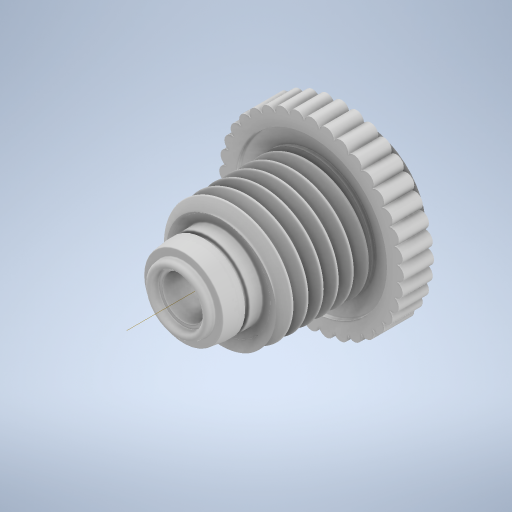
# Autodesk Inventor part: rosca
Saved by Autodesk Inventor 2024 (Build 280153000, 153)
## iProperties
Created: 2023-07-06
Part Number: rosca
Material: Genérico
Document SubType Name: Modeling
Designer: Arthur
Density: 1 g/cm^3
Appearance: Valor por defecto
Author: Arthur
## iProperties of the stored document rosca_3DPrint.ipt
Created: 2023-07-06
Part Number: rosca_3DPrint
Material: Genérico
Document SubType Name: Modeling
Designer: Arthur
Density: 1 g/cm^3
Appearance: Valor por defecto
Author: Arthur
Autodesk Inventor part; units mm, degrees
ref_plane "YZ Plane" through (0, 0, 0) normal (1, 0, 0) x (0, 1, 0)
ref_plane "XZ Plane" through (0, 0, 0) normal (0, 1, 0) x (-1, 0, 0)
ref_plane "XY Plane" through (0, 0, 0) normal (0, 0, 1) x (1, 0, 0)
sketch "Boceto1" plane through (0, 0, 0) normal (0, 0, 1) x (1, 0, 0)
  circle A0 centre (0, 0) radius 11.25
  arc A1 (0.999, 11.2056) -> (-0.999, 11.2056) centre (0, 11.25) ccw
  arc A2 (-0.962, 11.2088) -> (-2.9297, 10.8618) centre (-1.9535, 11.0791) ccw
  arc A3 (-2.8938, 10.8715) -> (-4.7713, 10.1881) centre (-3.8477, 10.5715) ccw
  arc A4 (-4.7376, 10.2038) -> (-6.4679, 9.2048) centre (-5.625, 9.7428) ccw
  arc A5 (-6.4375, 9.2261) -> (-7.9681, 7.9418) centre (-7.2314, 8.618) ccw
  arc A6 (-7.9418, 7.9681) -> (-9.2261, 6.4375) centre (-8.618, 7.2314) ccw
  arc A7 (-9.2048, 6.4679) -> (-10.2038, 4.7376) centre (-9.7428, 5.625) ccw
  arc A8 (-10.1881, 4.7713) -> (-10.8715, 2.8938) centre (-10.5715, 3.8477) ccw
  arc A9 (-10.8618, 2.9297) -> (-11.2088, 0.962) centre (-11.0791, 1.9535) ccw
  arc A10 (-11.2056, 0.999) -> (-11.2056, -0.999) centre (-11.25, 0) ccw
  arc A11 (-11.2088, -0.962) -> (-10.8618, -2.9297) centre (-11.0791, -1.9535) ccw
  arc A12 (-10.8715, -2.8938) -> (-10.1881, -4.7713) centre (-10.5715, -3.8477) ccw
  arc A13 (-10.2038, -4.7376) -> (-9.2048, -6.4679) centre (-9.7428, -5.625) ccw
  arc A14 (-9.2261, -6.4375) -> (-7.9418, -7.9681) centre (-8.618, -7.2314) ccw
  arc A15 (-7.9681, -7.9418) -> (-6.4375, -9.2261) centre (-7.2314, -8.618) ccw
  arc A16 (-6.4679, -9.2048) -> (-4.7376, -10.2038) centre (-5.625, -9.7428) ccw
  arc A17 (-4.7713, -10.1881) -> (-2.8938, -10.8715) centre (-3.8477, -10.5715) ccw
  arc A18 (-2.9297, -10.8618) -> (-0.962, -11.2088) centre (-1.9535, -11.0791) ccw
  arc A19 (-0.999, -11.2056) -> (0.999, -11.2056) centre (0, -11.25) ccw
  arc A20 (0.962, -11.2088) -> (2.9297, -10.8618) centre (1.9535, -11.0791) ccw
  arc A21 (2.8938, -10.8715) -> (4.7713, -10.1881) centre (3.8477, -10.5715) ccw
  arc A22 (4.7376, -10.2038) -> (6.4679, -9.2048) centre (5.625, -9.7428) ccw
  arc A23 (6.4375, -9.2261) -> (7.9681, -7.9418) centre (7.2314, -8.618) ccw
  arc A24 (7.9418, -7.9681) -> (9.2261, -6.4375) centre (8.618, -7.2314) ccw
  arc A25 (9.2048, -6.4679) -> (10.2038, -4.7376) centre (9.7428, -5.625) ccw
  arc A26 (10.1881, -4.7713) -> (10.8715, -2.8938) centre (10.5715, -3.8477) ccw
  arc A27 (10.8618, -2.9297) -> (11.2088, -0.962) centre (11.0791, -1.9535) ccw
  arc A28 (11.2056, -0.999) -> (11.2056, 0.999) centre (11.25, 0) ccw
  arc A29 (11.2088, 0.962) -> (10.8618, 2.9297) centre (11.0791, 1.9535) ccw
  arc A30 (10.8715, 2.8938) -> (10.1881, 4.7713) centre (10.5715, 3.8477) ccw
  arc A31 (10.2038, 4.7376) -> (9.2048, 6.4679) centre (9.7428, 5.625) ccw
  arc A32 (9.2261, 6.4375) -> (7.9418, 7.9681) centre (8.618, 7.2314) ccw
  arc A33 (7.9681, 7.9418) -> (6.4375, 9.2261) centre (7.2314, 8.618) ccw
  arc A34 (6.4679, 9.2048) -> (4.7376, 10.2038) centre (5.625, 9.7428) ccw
  arc A35 (4.7713, 10.1881) -> (2.8938, 10.8715) centre (3.8477, 10.5715) ccw
  arc A36 (2.9297, 10.8618) -> (0.962, 11.2088) centre (1.9535, 11.0791) ccw
  circle A37 centre (0, 0) radius 11.4037
  point P0 (-2.9515, 11.0151)
  point P1 (-4.8194, 10.3353)
  point P2 (-6.5409, 9.3414)
  point P3 (-8.0636, 8.0636)
  point P4 (-9.3414, 6.5409)
  point P5 (-10.3353, 4.8194)
  point P6 (-11.0151, 2.9515)
  point P7 (-11.3603, 0.9939)
  point P8 (-11.3603, -0.9939)
  point P9 (-11.0151, -2.9515)
  point P10 (-10.3353, -4.8194)
  point P11 (-9.3414, -6.5409)
  point P12 (-8.0636, -8.0636)
  point P13 (-6.5409, -9.3414)
  point P14 (-4.8194, -10.3353)
  point P15 (-2.9515, -11.0151)
  point P16 (-0.9939, -11.3603)
  point P17 (0.9939, -11.3603)
  point P18 (2.9515, -11.0151)
  point P19 (4.8194, -10.3353)
  point P20 (6.5409, -9.3414)
  point P21 (8.0636, -8.0636)
  point P22 (9.3414, -6.5409)
  point P23 (10.3353, -4.8194)
  point P24 (11.0151, -2.9515)
  point P25 (11.3603, -0.9939)
  point P26 (11.3603, 0.9939)
  point P27 (11.0151, 2.9515)
  point P28 (10.3353, 4.8194)
  point P29 (9.3414, 6.5409)
  point P30 (8.0636, 8.0636)
  point P31 (6.5409, 9.3414)
  point P32 (4.8194, 10.3353)
  point P33 (2.9515, 11.0151)
  point P34 (0.9939, 11.3603)
  point P35 (-0.9939, 11.3603)
  dimension "d1" = 22.5
  dimension "d4" = 360
  constraints: 75 point on circle, 38 centre point, 1 coincident, 145 other
  measures "d1" diameter of A0
extrude "Extrusión1" add sketch "Boceto1" along normal blind 4
sketch "Boceto2" plane through (0, 0, 0) normal (0, 0, -1) x (-1, 0, 0)
  circle A0 centre (0, 0) radius 8.25
  dimension "d8" = 16.5
  constraints: 1 centre point, 1 coincident
  measures "d8" diameter of A0
extrude "Extrusión2" add sketch "Boceto2" along normal blind 3
sketch "Boceto3" plane through (0, 0, 4) normal (0, 0, 1) x (1, 0, 0)
  circle A0 centre (0, 0) radius 8
  dimension "d11" = 16
  constraints: 1 centre point, 1 coincident
  measures "d11" diameter of A0
extrude "Extrusión3" add sketch "Boceto3" along normal blind 18
sketch "Boceto4" plane through (0, 0, 22) normal (0, 0, 1) x (1, 0, 0)
  circle A0 centre (0, 0) radius 8 projected
  circle A1 centre (0, 0) radius 5.5
  dimension "d14" = 11
  constraints: 1 centre point, 1 coincident
  measures "d14" diameter of A1
extrude "Extrusión4" cut sketch "Boceto4" against normal blind 6
sketch "Boceto5" plane through (0, 0, 22) normal (0, 0, 1) x (1, 0, 0)
  circle A0 centre (0, 0) radius 2.8
  dimension "d17" = 5.6
  constraints: 1 centre point, 1 coincident
  measures "d17" diameter of A0
extrude "Extrusión5" cut sketch "Boceto5" against normal blind 60
sketch "Boceto6" plane through (0, 0, 4) normal (0, 0, 1) x (1, 0, 0)
  circle A0 centre (0, 0) radius 10
  circle A1 centre (0, 0) radius 8
  circle A2 centre (0, 0) radius 8
  dimension "d20" = 20
  constraints: 3 centre point, 3 coincident
  measures "d20" diameter of A0
extrude "Extrusión6" cut sketch "Boceto6" against normal blind 0.5 contours A0 | A1
sketch "Boceto7" plane through (0, 0, 3.5) normal (0, 0, 1) x (1, 0, 0)
  circle A0 centre (0, 0) radius 8
  circle A1 centre (0, 0) radius 2.8
  constraints: 2 centre point, 2 coincident
extrude "Extrusión7" add sketch "Boceto7" along normal blind 0.5
sketch "Boceto8" plane through (0, 0, -3) normal (0, 0, -1) x (-1, 0, 0)
  circle A0 centre (0, 0) radius 2.8 projected
  circle A1 centre (0, 0) radius 5.4
  dimension "d27" = 10.8
  constraints: 1 centre point, 1 coincident
  measures "d27" diameter of A1
extrude "Extrusión8" cut sketch "Boceto8" against normal blind 10
fillet "Empalme1" radius 0.2 1 edges at (5.4, 0, 7)
fillet "Empalme2" radius 0.2 1 edges at (5.4, 0, -3)
fillet "Empalme3" radius 0.4 1 edges at (8.25, 0, 0)
thread "Rosca2" size "TR16x2" class "7e" standard "ISO Metric Trapezoidal Threads" length 12
sketch "Boceto10" plane through (0, 0, 16) normal (-1, 0, 0) x (0, 1, 0)
  line L0 (8, 0) -> (8, 12)
  line L1 (8, 12) -> (6.5171, 12)
  line L2 (6.5171, 12) -> (6.5171, 0)
  line L3 (6.5171, 0) -> (8, 0)
  line L4 (0, -2.4) -> (0, 14.4) projected
  constraints: 8 end point
revolve "Revolución1" cut sketch "Boceto10" angle 360 about axis through (0, 0, 16) along (0, 0, -1)
sketch "Boceto11" plane through (0, 0, 16) normal (-1, 0, 0) x (0, 1, 0)
  line L0 (8, 0) -> (8, 12)
  line L1 (8, 12) -> (6.5171, 12)
  line L2 (6.5171, 12) -> (6.5171, 0)
  line L3 (6.5171, 0) -> (8, 0)
  line L4 (0, -2.4) -> (0, 14.4) projected
  constraints: 8 end point
revolve "Revolución2" add sketch "Boceto11" angle 360 about axis through (0, 0, 16) along (0, 0, -1) separate body
sketch "Boceto9" plane through (0, 0, 16) normal (1, 0, 0) x (0, 0, -1)
  line L0 (-1.1668, -6.6184) -> (-1.0001, -6.6184) construction
  line L1 (0.1666, -7.899) -> (-0.0001, -8.2192) construction
  line L2 (-2.0001, -8.2192) -> (-2.1668, -7.899) construction
  line L3 (-0.8334, -6.6184) -> (-1.0001, -6.2982) construction
  line L4 (-1.0001, -6.2982) -> (-1.1668, -6.6184) construction
  line L5 (-2.0001, -8.2192) -> (-1.8334, -7.899) construction
  line L6 (-0.8334, -6.6184) -> (-0.1668, -7.899)
  line L7 (-2.1668, -7.899) -> (-1.8334, -7.899) construction
  arc A0 (-2.1668, -7.899) -> (-2.0001, -8.0002) centre (-2.0001, -7.8123) ccw construction
  line L8 (0.1666, -7.899) -> (-0.1668, -7.899) construction
  line L9 (-2.0001, -8.2192) -> (-2.0001, -7.899) construction
  line L10 (-0.0001, -8.2192) -> (-0.0001, -7.899) construction
  line L11 (-1.0001, -6.2982) -> (-1.0001, -6.5172) construction
  line L12 (-2.0001, -8.0002) -> (-0.0001, -8.0002)
  arc A1 (-2.0001, -8.0002) -> (-1.8334, -7.899) centre (-2.0001, -7.8123) ccw
  line L13 (-0.1668, -7.899) -> (-0.0001, -8.2192) construction
  line L14 (-1.8334, -7.899) -> (-1.1668, -6.6184)
  line L15 (-0.0001, -0.0002) -> (-0.0001, 0.0177)
  line L16 (-0.0001, 0.0177) -> (-0.0001, -0.0002)
  line L17 (-0.0001, -0.0002) -> (0.0334, -0.0002)
  arc A2 (-0.1668, -7.899) -> (-0.0001, -8.0002) centre (-0.0001, -7.8123) ccw
  arc A3 (-0.0001, -8.0002) -> (0.1666, -7.899) centre (-0.0001, -7.8123) ccw construction
  arc A4 (-1.0001, -6.5172) -> (-1.1668, -6.6184) centre (-1.0001, -6.7051) ccw
  arc A5 (-0.8334, -6.6184) -> (-1.0001, -6.5172) centre (-1.0001, -6.7051) ccw
  line L18 (-1.0001, -6.5172) -> (-1.0001, -6.6184) construction
  line L19 (-1.0001, -6.6184) -> (-0.8334, -6.6184) construction
  dimension "d35" = 55
  dimension "d36" = 0.3202
  dimension "d37" = 0.3202
  dimension "Boceto9_ThreadOffset" = 0
  dimension "Boceto9_MajorRadius" = 8
  dimension "d40" = 2
  dimension "Boceto9_MinorRadius" = 6.5171
  constraints: 40 end point, 12 point on circle, 10 parallel, 8 tangent, 6 centre point, 6 collinear, 2 midpoint, 2 point on line, 1 horizontal, 1 perpendicular, 3 other
  measures "d35" angle of L6 L14
  measures "d36" distance of L3.end L0.end
  measures "d37" distance of L1.end L10.end
  measures "Boceto9_ThreadOffset" distance between parallel lines of L15 L10
  measures "Boceto9_MajorRadius" distance from line of L12 L15.start
  measures "d40" distance from line of L1.end L9
  measures "Boceto9_MinorRadius" distance edge to line of A5 L17
coil "Bobina1" sketch "Boceto9" operation cut axis through (0, 0, 16) along (0, 0, -1) pitch 2.002 turns 7.992008 hand right bodies 2
sketch "Boceto12" plane through (0, 0, 22) normal (0, 0, 1) x (1, 0, 0)
  circle A0 centre (0, 0) radius 2.8 projected
  circle A1 centre (0, 0) radius 5.5 projected
  circle A2 centre (0, 0) radius 4.25
  circle A3 centre (0, 0) radius 3.25
  dimension "d54" = 8.5
  dimension "d55" = 6.5
  constraints: 2 centre point, 2 coincident
  measures "d54" diameter of A2
  measures "d55" diameter of A3
extrude "Extrusión9" cut sketch "Boceto12" against normal blind 1 bodies 1
fillet "Empalme4" radius 0.5 2 edges at (-4.25, 0, 22) (-3.25, 0, 22)
sketch "Boceto13" plane through (0, 0, 0) normal (1, 0, 0) x (0, 1, 0)
  line L0 (-5.5, 21) -> (5.5, 21) projected
  line L1 (5.5, 16) -> (-5.5, 16) projected
  line L2 (5.5, 21) -> (5.5, 19)
  line L3 (5.5, 16) -> (5.5, 21) projected
  line L4 (5.5, 21) -> (5.25, 21)
  line L5 (5.25, 21) -> (5.5, 19)
  line L6 (5.5, 21) -> (5.5, 18)
  line L7 (5.5, 18) -> (5.5, 18.5)
  line L8 (5.5, 18.5) -> (5.5, 17.5)
  line L9 (5, 17.875) -> (5, 18.125)
  line L10 (0, -4.2) -> (0, 25.2) projected
  line L11 (5.5, 18) -> (5.5, 18.25)
  line L12 (5.5, 16) -> (5.5, 21) projected
  line L13 (5.5, 18.25) -> (5.125, 18.25)
  line L14 (5.5, 17.5) -> (5.5, 17.75)
  line L15 (5.5, 16) -> (5.5, 21) projected
  line L16 (5.125, 17.75) -> (5.5, 17.75)
  arc A0 (5.125, 18.25) -> (5, 18.125) centre (5.125, 18.125) ccw
  arc A1 (5, 17.875) -> (5.125, 17.75) centre (5.125, 17.875) ccw
  point P0 (0, 0)
  point P1 (5.25, 17.5)
  dimension "d59" = 2
  dimension "d60" = 0.25
  constraints: 22 end point, 6 point on line, 4 point on circle, 4 tangent, 2 centre point, 2 perpendicular, 2 other
  measures "d59" distance of L0.end L2.end
  measures "d60" distance of L3.end L4.end
revolve "Revolución3" cut sketch "Boceto13" angle 360 about axis through (0, 0, -10) along (0, 0, 1) bodies 1 contours L0 L2 L5 | L3 L16 A1 L9 A0 L13
fillet "Empalme5" radius 0.1 2 edges at (-5.5, 0, 18.25) (-5.5, 0, 17.75)
fillet "Empalme6" radius 0.1 1 edges at (0, -5.25, 21)
fillet "Empalme7" radius 0.1 1 edges at (-4.25, 0, 21)
fillet "Empalme8" radius 0.1 1 edges at (-5.5, 0, 16)
fillet "Empalme9" radius 0.1 1 edges at (8.25, 0, -3)
fillet "Empalme10" radius 0.1 1 edges at (-10, 0, 3.5)
equation "\"d35\" = d42"
equation "\"d36\" = 0.160083 * Boceto9_Pitch"
equation "\"d37\" = 0.160083 * Boceto9_Pitch"
equation "\"d40\" = Boceto9_Pitch"
equation "\"d42\" = 55deg"
equation "\"Boceto9_Pitch\" = 2"
